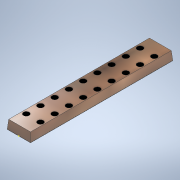
# Autodesk Inventor part: VeroBoardLeadsSIngleHeater
Saved by Autodesk Inventor 2021 (Build 250183000, 183)
## iProperties
Created: 2021-12-15
Part Number: VeroBoardLeadsSIngleHeater
Material: Generic
Document SubType Name: Sheet Metal
Designer: Unit-005
Density: 1 g/cm^3
Sheet Metal Rule: Default
Appearance: Cardboard
Author: Unit-005
Autodesk Inventor part; units mm, degrees
ref_plane "YZ Plane" through (0, 0, 0) normal (1, 0, 0) x (0, 1, 0)
ref_plane "XZ Plane" through (0, 0, 0) normal (0, 1, 0) x (-1, 0, 0)
ref_plane "XY Plane" through (0, 0, 0) normal (0, 0, 1) x (1, 0, 0)
sketch "Sketch1" plane through (0, 0, 0) normal (0, 0, 1) x (1, 0, 0)
  point P0 (0, 0)
sketch "Sketch2" plane through (0, 0, 0) normal (0, 1, 0) x (-1, 0, 0)
  line L0 (2.87, 0) -> (-2.87, 0) projected
  line L1 (0, -30) -> (0, 5) projected
  line L2 (2.05, 0) -> (-2.05, 0)
  line L3 (-2.05, 0) -> (-2.05, -25)
  line L4 (-2.05, -25) -> (2.05, -25)
  line L5 (2.05, -25) -> (2.05, 0)
  point P0 (0, 0)
  dimension "d0" = 4.1
  dimension "d1" = 25
  constraints: 8 end point, 2 parallel, 1 horizontal, 1 perpendicular, 1 point on line, 1 other
  measures "d0" distance of L4.end L3.end
  measures "d1" distance of L3.end L2.end
sketch "Sketch2 outline for Extrusion1" plane through (0, 0, 0) normal (0, 1, 0) x (-1, 0, 0)
  line L0 (2.05, -25) -> (2.05, 0)
  line L1 (-2.05, -25) -> (2.05, -25)
  line L2 (-2.05, 0) -> (-2.05, -25)
  line L3 (2.05, 0) -> (-2.05, 0)
extrude "Extrusion1" add sketch "Sketch2 outline for Extrusion1" along normal blind 1.5 draft -5
sketch "Sketch3" plane through (0, 0, 0) normal (0, -1, 0) x (1, 0, 0)
  line L0 (-2.05, 0) -> (2.05, 0) projected
  line L1 (-2.05, -25) -> (-2.05, 0) projected
  line L2 (2.05, -25) -> (-2.05, -25) projected
  line L3 (2.05, 0) -> (2.05, -25) projected
  line L4 (-2.87, 0) -> (2.87, 0) projected
  line L5 (0, -30) -> (0, 5) projected
  line L6 (-2.05, 0) -> (2.05, 0) projected
  line L7 (2.05, 0) -> (0.25, 0)
  line L8 (0.25, 0) -> (0.25, -25)
  line L9 (0.25, -25) -> (2.05, -25)
  line L10 (2.05, -25) -> (2.05, 0)
  point P0 (0, 0)
  point P1 (0.25, 0)
  dimension "d4" = 1.8
  constraints: 8 end point, 2 parallel, 1 horizontal, 1 perpendicular, 1 point on line
  measures "d4" distance of L9.end L8.end
extrude "Extrusion2" add sketch "Sketch3" along normal blind 0.035 contours L0 L3 L2 L8
mirror "Mirror1" about plane through (0, 0, 0) normal (1, 0, 0) of "Extrusion2"
sketch "Sketch4" plane through (0, -0.035, 0) normal (0, -1, 0) x (1, 0, 0)
  circle A0 centre (1.3, -2.5) radius 0.5
  line L0 (2.05, 0) -> (0.25, 0) projected
  line L1 (2.05, -25) -> (2.05, 0) projected
  point P0 (0, 0)
  dimension "d7" = 1
  dimension "d8" = 2.5
  dimension "d9" = 0.75
  constraints: 1 centre point
  measures "d7" diameter of A0
  measures "d8" distance from line of L0 A0.centre
  measures "d9" distance from line of L1 A0.centre
extrude "Extrusion3" cut sketch "Sketch4" against normal through all
pattern_linear "Rectangular Pattern1" count 9 spacing 2.5 along (0, 0, -1) count 2 spacing 2.5 along (-1, 0, 0) of "Extrusion3"
equation "\"BendRadius\" = Thickness"
equation "\"BendReliefWidth\" = Thickness"
equation "\"BendReliefDepth\" = 0.5 * Thickness"
equation "\"CornerReliefSize\" = 4 * Thickness"
equation "\"MinimumRemnant\" = 2 * Thickness"
equation "\"TransitionRadius\" = BendRadius"
equation "\"JacobiRadiusSize\" = BendRadius"
equation "\"GapSize\" = Thickness"
equation "\"Thickness\" = 3.048"
body "Solid1"
